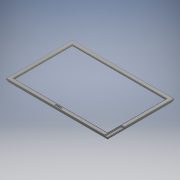
# Autodesk Inventor part: OBUDOWA PRZEDNIA
Saved by Autodesk Inventor 2017 SP1 (Build 210196100, 196)
## iProperties
Created: 2021-03-07
Part Number: OBUDOWA PRZEDNIA
Material: Tworzywo sztuczne, nieprzezroczyste czarne
Document SubType Name: Modeling
Designer: Administrator
Density: 0.952 g/cm^3
Appearance: Teksturowany - szary
Author: Administrator
Autodesk Inventor part; units mm, degrees
ref_plane "YZ Plane" through (0, 0, 0) normal (1, 0, 0) x (0, 1, 0)
ref_plane "XZ Plane" through (0, 0, 0) normal (0, 1, 0) x (-1, 0, 0)
ref_plane "XY Plane" through (0, 0, 0) normal (0, 0, 1) x (1, 0, 0)
sketch "Szkic1" plane through (0, 0, 0) normal (0, 0, 1) x (1, 0, 0)
  line L0 (-218.2, 284.6) -> (218.2, 284.6)
  line L1 (219.2, 283.6) -> (219.2, 0.3)
  line L2 (218.2, -0.7) -> (-218.2, -0.7)
  line L3 (-219.2, 0.3) -> (-219.2, 283.6)
  arc A0 (219.2, 283.6) -> (218.2, 284.6) centre (218.2, 283.6) ccw
  arc A1 (-218.2, 284.6) -> (-219.2, 283.6) centre (-218.2, 283.6) ccw
  arc A2 (-219.2, 0.3) -> (-218.2, -0.7) centre (-218.2, 0.3) ccw
  arc A3 (218.2, -0.7) -> (219.2, 0.3) centre (218.2, 0.3) ccw
  line L4 (214.5, 280.9) -> (-214.5, 280.9)
  line L5 (-215.5, 279.9) -> (-215.5, 3.3625)
  line L6 (-214.5, 2.3625) -> (214.5, 2.3625)
  line L7 (215.5, 3.3625) -> (215.5, 279.9)
  arc A4 (-214.5, 280.9) -> (-215.5, 279.9) centre (-214.5, 279.9) ccw
  arc A5 (215.5, 279.9) -> (214.5, 280.9) centre (214.5, 279.9) ccw
  arc A6 (214.5, 2.3625) -> (215.5, 3.3625) centre (214.5, 3.3625) ccw
  arc A7 (-215.5, 3.3625) -> (-214.5, 2.3625) centre (-214.5, 3.3625) ccw
  point P0 (0, 0)
  point P1 (219.2, 284.6)
  point P2 (-219.2, -0.7)
  point P3 (219.2, -0.7)
  dimension "d7" = 1
  constraints: 16 end point, 16 point on circle, 16 tangent, 8 centre point, 6 equal radius, 4 parallel, 2 horizontal, 2 perpendicular
  measures "d7" radius of A4
extrude "Wyciągnięcie proste1" add sketch "Szkic1" along normal blind 1.5
sketch "Szkic2" plane through (0, 0, 0) normal (0, 0, -1) x (-1, 0, 0)
  line L0 (217, 2.5) -> (217, 281.4)
  line L1 (216, 282.4) -> (-216, 282.4)
  line L2 (-217, 281.4) -> (-217, 2.5)
  line L3 (-215.5, 3.3625) -> (-215.5, 279.9)
  arc A0 (-214.5, 280.9) -> (-215.5, 279.9) centre (-214.5, 279.9) ccw
  line L4 (-214.5, 280.9) -> (214.5, 280.9)
  arc A1 (215.5, 279.9) -> (214.5, 280.9) centre (214.5, 279.9) ccw
  line L5 (215.5, 279.9) -> (215.5, 3.3625)
  arc A2 (214.5, 2.3625) -> (215.5, 3.3625) centre (214.5, 3.3625) ccw
  line L6 (216, 1.5) -> (73, 1.5)
  line L7 (214.5, 2.3625) -> (-214.5, 2.3625)
  arc A3 (-215.5, 3.3625) -> (-214.5, 2.3625) centre (-214.5, 3.3625) ccw
  line L8 (-51.8, 1.5) -> (-216, 1.5)
  line L9 (-216, 282.4) -> (-215.9969, 282.4)
  line L10 (-39.9, 1.5) -> (-51.8, 1.5)
  line L11 (61.1, 1.5) -> (-39.9, 1.5)
  line L12 (73, 1.5) -> (61.1, 1.5)
  arc A4 (-216, 282.4) -> (-217, 281.4) centre (-216, 281.4) ccw
  arc A5 (217, 281.4) -> (216, 282.4) centre (216, 281.4) ccw
  arc A6 (216, 1.5) -> (217, 2.5) centre (216, 2.5) ccw
  arc A7 (-217, 2.5) -> (-216, 1.5) centre (-216, 2.5) ccw
  point P0 (0, 0)
  dimension "d10" = 1
  dimension "d11" = 1
  dimension "d12" = 1
  dimension "d13" = 1
  constraints: 26 end point, 16 point on circle, 8 centre point, 6 tangent, 1 point on line
  measures "d10" radius of A4
  measures "d11" radius of A5
  measures "d12" radius of A6
  measures "d13" radius of A7
extrude "Wyciągnięcie proste2" add sketch "Szkic2" along normal blind 5
sketch "Szkic3" plane through (0, 0, 1.5) normal (0, 0, 1) x (1, 0, 0)
  line L0 (-220.2, 284.6) -> (-220.2, -0.7) projected
  arc A0 (-220.2, -0.7) -> (-219.2, -1.7) centre (-219.2, -0.7) ccw
  line L1 (-219.2, -1.7) -> (219.2, -1.7) projected
  arc A1 (-219.2, 285.6) -> (-220.2, 284.6) centre (-219.2, 284.6) ccw
  line L2 (219.2, 285.6) -> (-219.2, 285.6) projected
  arc A2 (220.2, 284.6) -> (219.2, 285.6) centre (219.2, 284.6) ccw
  line L3 (220.2, -0.7) -> (220.2, 284.6) projected
  arc A3 (219.2, -1.7) -> (220.2, -0.7) centre (219.2, -0.7) ccw
  line L4 (-204.2, 269.6) -> (204.2, 269.6)
  line L5 (204.2, 269.6) -> (204.2, 14.3)
  line L6 (204.2, 14.3) -> (-204.2, 14.3)
  line L7 (-204.2, 14.3) -> (-204.2, 269.6)
  point P0 (0, 0)
  constraints: 8 end point, 8 point on circle, 4 centre point, 2 parallel, 1 horizontal, 1 perpendicular
extrude "Wyciągnięcie proste4" add sketch "Szkic3" along normal blind 5.2
fillet "Zaokrąglenie2" radius 0.5 8 edges at (-219.9071, 285.3071, 1.5) (-220.2, 141.95, 1.5) (-219.9071, -1.4071, 1.5) (0, -1.7, 1.5) (219.9071, -1.4071, 1.5) (220.2, 141.95, 1.5) (219.9071, 285.3071, 1.5) (0, 285.6, 1.5)
fillet "Zaokrąglenie3" radius 1 8 edges at (-219.9071, 285.3071, 6.7) (-220.2, 141.95, 6.7) (-219.9071, -1.4071, 6.7) (0, -1.7, 6.7) (219.9071, -1.4071, 6.7) (220.2, 141.95, 6.7) (219.9071, 285.3071, 6.7) (0, 285.6, 6.7)
sketch "Szkic4" plane through (0, 0, 1.5) normal (0, 0, -1) x (-1, 0, 0)
  line L0 (-215.5, 3.3625) -> (-215.5, 279.9) projected
  arc A0 (-214.5, 280.9) -> (-215.5, 279.9) centre (-214.5, 279.9) ccw projected
  line L1 (-204.2, 14.3) -> (-204.2, 269.6) projected
  line L2 (-204.2, 269.6) -> (204.2, 269.6) projected
  line L3 (-214.5, 280.9) -> (214.5, 280.9) projected
  line L4 (204.2, 269.6) -> (204.2, 14.3) projected
  arc A1 (215.5, 279.9) -> (214.5, 280.9) centre (214.5, 279.9) ccw projected
  line L5 (215.5, 279.9) -> (215.5, 3.3625) projected
  line L6 (204.2, 14.3) -> (-204.2, 14.3) projected
  line L7 (214.5, 2.3625) -> (-214.5, 2.3625) projected
  arc A2 (214.5, 2.3625) -> (215.5, 3.3625) centre (214.5, 3.3625) ccw projected
  arc A3 (-215.5, 3.3625) -> (-214.5, 2.3625) centre (-214.5, 3.3625) ccw projected
  point P0 (0, 0)
extrude "Wyciągnięcie proste5" add sketch "Szkic4" along normal blind 1.1
chamfer "Faza1" distance 1.5 distance2 1 1 edges at (-204.2, 141.95, 6.7) measured on face at (68.0667, 4.3, 6.7)
chamfer "Faza2" distance 1.5 distance2 1 1 edges at (0, 269.6, 6.7) measured on face at (68.0667, 4.3, 6.7)
chamfer "Faza3" distance 1.5 distance2 1 1 edges at (204.2, 141.95, 6.7) measured on face at (68.0667, 4.3, 6.7)
chamfer "Faza4" distance 1.5 distance2 1 1 edges at (0, 14.3, 6.7) measured on face at (68.0667, 4.3, 6.7)
sketch "Szkic5" plane through (0, 0, 6.7) normal (0, 0, 1) x (1, 0, 0)
  line L0 (219.2, -1.7) -> (206.2, -1.7)
  line L1 (206.2, -1.7) -> (206.45, -1.7)
  line L2 (206.2, 71.425) -> (220.2, 71.425)
  line L3 (220.2, 71.425) -> (220.2, -0.7)
  arc A0 (219.2, -1.7) -> (220.2, -0.7) centre (219.2, -0.7) ccw
  line L4 (206.2, -1.7) -> (206.2, 71.425)
  constraints: 10 end point, 2 point on circle, 1 centre point, 1 horizontal, 1 point on line
extrude "Wyciągnięcie proste6" cut sketch "Szkic5" against normal blind 6.2
sketch "Szkic6" plane through (0, 0, 6.7) normal (0, 0, 1) x (1, 0, 0)
  line L0 (2.6567, 2.6528) -> (2.657, 4.8393)
  line L1 (-6.8758, 5.3818) -> (-2.1024, 2.2136)
  line L2 (-2.2336, 10.8259) -> (-6.9572, 7.6927)
  line L3 (-2.1024, 2.2136) -> (2.6564, 5.385)
  line L4 (14.4188, 2.6234) -> (14.4191, 4.8375)
  line L5 (1.9087, 8.0765) -> (-1.7626, 5.6414)
  line L6 (1.9087, 8.0765) -> (0.1103, 9.2702)
  line L7 (0.1103, 9.2702) -> (-3.5698, 6.8293)
  line L8 (-3.5698, 6.8293) -> (-4.1314, 7.2021)
  line L9 (-4.1314, 7.2021) -> (-0.4514, 9.643)
  line L10 (-0.4514, 9.643) -> (-2.2336, 10.8259)
  line L11 (14.4188, 2.6234) -> (14.4188, 2.652)
  line L12 (2.6564, 2.6222) -> (2.6564, 5.385)
  line L13 (8.7309, 2.6234) -> (8.7309, 10.6234)
  line L14 (8.7309, 10.6234) -> (11.5831, 10.6234)
  line L15 (8.7309, 10.6234) -> (11.5831, 10.6234)
  line L16 (11.5831, 10.6234) -> (11.5831, 4.8379)
  line L17 (11.5831, 4.8379) -> (14.4191, 4.8375)
  line L18 (14.4188, 2.6234) -> (8.7309, 2.6234)
  line L19 (8.3444, 2.623) -> (2.6564, 2.623)
  line L20 (8.3444, 2.623) -> (8.3447, 4.8375)
  line L21 (5.5087, 4.8379) -> (8.3447, 4.8375)
  line L22 (5.5087, 10.6234) -> (5.5087, 4.8379)
  line L23 (2.6567, 10.6234) -> (5.5087, 10.6234)
  line L24 (2.8855, 10.652) -> (2.5712, 10.652)
  line L25 (2.6564, 2.623) -> (2.6564, 5.385)
  line L26 (2.6567, 7.7426) -> (2.6567, 10.6234)
  line L27 (-14.4194, 2.4022) -> (-14.4194, 10.4022)
  line L28 (-14.4194, 10.4022) -> (-10.5724, 10.4022)
  line L29 (-14.4194, 10.4022) -> (-10.5724, 10.4022)
  line L30 (-14.4194, 2.4022) -> (-10.5724, 2.4022)
  arc A0 (-10.5724, 2.4022) -> (-6.8758, 5.3818) centre (-10.7474, 6.4022) ccw
  arc A1 (-6.9572, 7.6927) -> (-10.5724, 10.4022) centre (-10.7474, 6.4022) ccw
  line L31 (-11.568, 4.7844) -> (-11.568, 7.9195)
  line L32 (-11.568, 7.9195) -> (-10.9818, 7.9195)
  arc A2 (-10.9818, 4.7844) -> (-10.9818, 7.9195) centre (-10.9818, 6.352) ccw
  line L33 (-7.0718, 7.99) -> (-7.0718, 7.9899)
  line L34 (-1.1458, 5.2204) -> (-1.7626, 5.6414)
  line L35 (-1.1458, 5.2204) -> (2.6567, 7.7426)
  line L36 (-11.568, 4.7844) -> (-10.9818, 4.7844)
  constraints: 76 end point, 7 point on circle, 6 horizontal, 3 centre point, 2 collinear, 2 perpendicular, 1 point on line, 1 tangent, 1 vertical
extrude "Wyciągnięcie proste7" cut sketch "Szkic6" against normal blind 0.01
